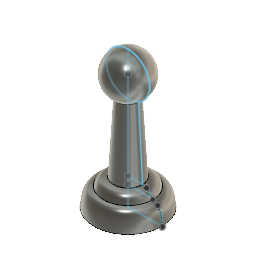
verkefni3 (Autodesk Fusion 360 design; units mm, degrees)
Autodesk Fusion 360 part; units mm, degrees
note: some values were not read from the file. Set by a fixed rule: which sketch regions a step uses.
sketch "Sketch1" plane through (0, 0, 0) normal (0, 1, 0) x (1, 0, 0)
  line L0 (50, 0) -> (50, -60)
  circle A0 centre (50, -50.491) radius 9.509
  line L1 (50, 0) -> (65, 0)
  spline S0 degree 5 poles (50, -8.5443) (50.8286, -8.5351) (52.4081, -8.5175) (54.5436, -8.4933) (56.941, -8.4553) (59.2768, -8.3388) (61.0591, -8.0737) (62.3952, -7.5752) (63.3805, -6.7678) (64.092, -5.609) (64.5852, -4.098) (64.8334, -2.6187) (64.9452, -1.3647) (64.9871, -0.4654) (65, 0) knots 0 0 0 0 0 0 0.1 0.2 0.3 0.4 0.5 0.6 0.7 0.8 0.9 1 1 1 1 1 1
  line L2 (46, -8.5886) -> (54, -8.5)
  spline S1 degree 5 poles (50, -11.7732) (50.381, -11.7738) (51.126, -11.7752) (52.1924, -11.7782) (53.5127, -11.7794) (54.996, -11.7491) (56.3123, -11.6507) (57.4598, -11.4453) (58.4369, -11.0976) (59.247, -10.587) (59.9016, -9.9122) (60.3106, -9.2461) (60.5567, -8.679) (60.6943, -8.2714) (60.7565, -8.0603) knots 0 0 0 0 0 0 0.1 0.2 0.3 0.4 0.5 0.6 0.7 0.8 0.9 1 1 1 1 1 1
  line L3 (48.2485, -11.7706) -> (51.7515, -11.7758)
  line L4 (56.3534, -11.6132) -> (54.6267, -42.1835)
  point P0 (63, -7)
  point P1 (58.1447, -11.1686)
  constraint vertical L0
  constraint coincident L0 A0.centre
  constraint coincident L0.end A0
  constraint perpendicular L0 L1
  constraint coincident L0 S0.start
  constraint midpoint S0.start L2
  constraint coincident L0 S1.start
  constraint coincident S0 S1.end
  constraint midpoint S1.start L3
  constraint coincident S1 L4.start
  constraint coincident A0 L4.end
revolve "Revolve1" add sketch "Sketch1" angle 360 about axis through (50, 0, 0) along (0, 0, 1) contours L0 L1 S0 | L0 S0 S1 L3 | L0 A0 S1 L3 L4 | L0 A0 picked at (52.8975, -48.5628)
